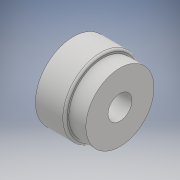
# Autodesk Inventor part: plunger_adaptor2
Saved by Autodesk Inventor 2018 (Build 220112000, 112)
## iProperties
Created: 2017-10-07
Part Number: plunger_adaptor2
Material: Generic
Document SubType Name: Modeling
Designer: MISAKA
Density: 1 g/cm^3
Appearance: Default
Author: MISAKA
Autodesk Inventor part; units mm, degrees
ref_plane "YZ Plane" through (0, 0, 0) normal (1, 0, 0) x (0, 1, 0)
ref_plane "XZ Plane" through (0, 0, 0) normal (0, 1, 0) x (-1, 0, 0)
ref_plane "XY Plane" through (0, 0, 0) normal (0, 0, 1) x (1, 0, 0)
sketch "Sketch1" plane through (0, 0, 0) normal (0, 1, 0) x (-1, 0, 0)
  line L0 (16.8, 0) -> (-2.8, 0) projected
  line L1 (0, -10.632) -> (0, 1.772) projected
  line L2 (14, 0) -> (10.9, -8.86)
  line L3 (10.9, -8.86) -> (4, -8.86)
  line L4 (4, -8.86) -> (4, -7.96)
  line L5 (4, -7.96) -> (0, -7.96)
  line L6 (14, 0) -> (9, 0)
  line L7 (0, -7.96) -> (0, -2.8)
  line L8 (9, 0) -> (9, -2.8)
  line L9 (9, -2.8) -> (0, -2.8)
  point P0 (0, 0)
  dimension "d0" = 5.6
  dimension "d1" = 14
  dimension "d2" = 17.72
  dimension "d3" = 15.92
  dimension "d4" = 9
  dimension "d5" = 4
  dimension "d6" = 3.1
  dimension "d7" = 6.9
  constraints: 16 end point, 4 perpendicular, 2 collinear, 2 point on line, 1 horizontal
  measures "d0" diameter of L9 L0
  measures "d1" distance from line of L2.start L1
  measures "d2" diameter of L3 L0
  measures "d3" diameter of L5 L0
  measures "d4" distance between parallel lines of L8 L1
  measures "d5" distance between parallel lines of L4 L1
  measures "d6" horizontal distance of L2.end L2.start
  measures "d7" distance of L3.end L2.end
revolve "Revolution1" add sketch "Sketch1" angle 360 about axis through (-10, 0, 0) along (1, 0, 0) contours L2 L3 L4 L5 L1 L9 L8 L0
fillet "Fillet1" radius 0.5 1 edges at (-4, 0, 8.86)
body "Solid1"
